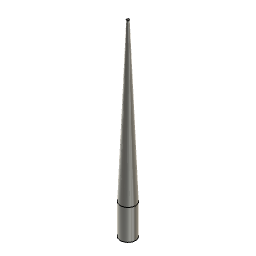
single_tip_press_fit (Autodesk Fusion 360 design; units mm, degrees)
Autodesk Fusion 360 part; units mm, degrees
sketch "Sketch1" plane through (0, 0, 0) normal (0, 0, 1) x (1, 0, 0)
  circle A0 centre (0, 0) radius 1.5875
  dimension "d1" = 3.175
  constraint coincident A0.centre origin
  measures "d1" diameter of A0
ref_plane "WorkPlane1" through (0, 0, 33.02) normal (0, 0, 1) x (1, 0, 0)
sketch "Sketch2" plane through (0, 0, 33.02) normal (0, 0, 1) x (1, 0, 0)
  circle A0 centre (0, 0) radius 0.254
  dimension "d3" = 0.508
  constraint coincident A0.centre origin
  measures "d3" diameter of A0
loft "Loft1" add profiles "Sketch1", "Sketch2" section 1 section 2
extrude "Extrude2" add 1 faces at (-0.3879, 0.3599, 0) along direction (0, 0, -1) blind 6.35
sketch "Sketch4" plane through (0, 0, 0) normal (0, 1, 0) x (1, 0, 0)
equation "d1 = ( 1 / 8 ) * 1 in"
